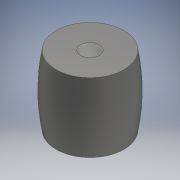
# Autodesk Inventor part: Roller
Saved by Autodesk Inventor 2017.3 (Build 213257000, 257)
## iProperties
Created: 2020-07-21
Part Number: Roller
Material: Generic
Document SubType Name: Modeling
Designer: Fahar Endra
Density: 1 g/cm^3
Appearance: Default
Author: Fahar Endra
Autodesk Inventor part; units mm, degrees
ref_plane "YZ Plane" through (0, 0, 0) normal (1, 0, 0) x (0, 1, 0)
ref_plane "XZ Plane" through (0, 0, 0) normal (0, 1, 0) x (-1, 0, 0)
ref_plane "XY Plane" through (0, 0, 0) normal (0, 0, 1) x (1, 0, 0)
sketch "Sketch1" plane through (0, 0, 0) normal (1, 0, 0) x (0, 1, 0)
  arc A0 (49.1369, -9.25) -> (49.1369, 9.25) centre (0, 0) ccw
  line L0 (40.0685, 9.25) -> (49.1369, 9.25)
  line L1 (40.0685, -9.25) -> (49.1369, -9.25)
  line L2 (40.0685, 9.25) -> (40.0685, -9.25)
  constraints: 6 end point, 2 point on circle, 1 centre point, 1 coincident
revolve "Revolution1" add sketch "Sketch1" angle 360 about axis through (0, 40.0685, 9.25) along (0, 0, -1)
hole "Hole1" at (0, 40.0685, 9.25) direction (0, 0, -1) diameter 5 end through all
body "Solid1"
